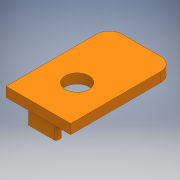
# Autodesk Inventor part: Rotary Encoder Mount Mk2
Saved by Autodesk Inventor 2018 (Build 220112000, 112)
## iProperties
Created: 2018-01-13
Part Number: Rotary Encoder Mount Mk2
Material: Generic
Document SubType Name: Modeling
Designer: Moochster
Density: 1 g/cm^3
Appearance: Orange
Mass: 1.86034 g
Surface Area: 16.5781 cm^2
Volume: 1.86034 cm^3
Author: Moochster
Autodesk Inventor part; units mm, degrees
ref_plane "YZ Plane" through (0, 0, 0) normal (1, 0, 0) x (0, 1, 0)
ref_plane "XZ Plane" through (0, 0, 0) normal (0, 1, 0) x (-1, 0, 0)
ref_plane "XY Plane" through (0, 0, 0) normal (0, 0, 1) x (1, 0, 0)
sketch "Sketch1" plane through (0, 0, 0) normal (0, 0, 1) x (1, 0, 0)
  line L0 (-10, -12) -> (10, -12)
  line L1 (10, -12) -> (10, 20)
  line L2 (10, 20) -> (-10, 20)
  line L3 (-10, 20) -> (-10, -12)
  line L4 (6.3, -6.7) -> (-6.3, -6.7) construction
  line L5 (6.3, 6.7) -> (6.3, -6.7) construction
  line L6 (-6.3, 6.7) -> (6.3, 6.7) construction
  line L7 (-6.3, -6.7) -> (-6.3, 6.7) construction
  line L8 (6.45, -6.85) -> (-6.45, -6.85)
  line L9 (-6.45, -6.85) -> (-6.45, 6.85)
  line L10 (-6.45, 6.85) -> (6.45, 6.85)
  line L11 (6.45, 6.85) -> (6.45, -6.85)
  circle A0 centre (0, 0) radius 3.535 construction
  circle A1 centre (0, 0) radius 3.685
  line L12 (4.65, -11.15) -> (-4.65, -11.15) construction
  line L13 (-4.65, -11.15) -> (-4.65, -8.85) construction
  line L14 (-4.65, -8.85) -> (4.65, -8.85) construction
  line L15 (4.65, -8.85) -> (4.65, -11.15) construction
  line L16 (4.5, -9) -> (-4.5, -9)
  line L17 (-4.5, -9) -> (-4.5, -11)
  line L18 (-4.5, -11) -> (4.5, -11)
  line L19 (4.5, -11) -> (4.5, -9)
  point P0 (0, 20)
  point P1 (0, 6.85)
  point P2 (6.45, 0)
  point P3 (0, -8.85)
  point P4 (0, -9)
  point P5 (0, -11)
  point P6 (0, -11.15)
  point P7 (0, -12)
  dimension "d0" = 20
  dimension "d1" = 32
  dimension "d2" = 0.15
  dimension "d3" = 0.15
  dimension "d5" = 7.07
  dimension "d6" = 12.9
  dimension "d7" = 13.7
  dimension "d8" = 20
  dimension "d18" = 2
  dimension "d19" = 2.3
  dimension "d20" = 9
  dimension "d21" = 9.3
  dimension "d22" = 0.85
  constraints: 40 end point, 8 midpoint, 5 vertical alignment, 3 horizontal, 2 centre point, 2 coincident, 2 parallel, 2 vertical, 1 horizontal alignment, 1 perpendicular, 6 other
  measures "d0" distance of L1.end L2.end
  measures "d1" distance of L0.end L1.end
  measures "d2" distance between parallel lines of L5 L11
  measures "d3" radial gap between concentric circles of A0 A1
  measures "d5" diameter of A0
  measures "d6" distance of L9.end L10.end
  measures "d7" distance of L10.end L8.start
  measures "d8" distance from line of A0.centre L2
  measures "d18" distance of L18.end L16.start
  measures "d19" distance of L14.end L12.start
  measures "d20" distance of L16.start L16.end
  measures "d21" distance of L13.end L14.end
  measures "d22" distance between parallel lines of L0 L12
extrude "Extrusion1" add sketch "Sketch1" along normal blind 3 contours L3 L2 L1 L0 | L19 L18 L17 L16
extrude "Extrusion2" add sketch "Sketch1" along normal blind 3 contours L8 L9 L10 L11
fillet "Fillet1" radius 4 2 edges at (10, 20, 1.5) (-10, 20, 1.5)
extrude "Extrusion3" add sketch "Sketch1" against normal blind 5 contours L19 L18 L17 L16
fillet "Fillet2" radius 0.5 4 edges at (4.5, -9, -2.5) (4.5, -11, -2.5) (-4.5, -9, -2.5) (-4.5, -11, -2.5)
body "Solid1"
